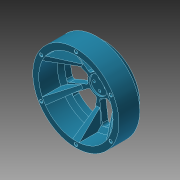
# Autodesk Inventor part: Переходник
Saved by Autodesk Inventor 2022 (Build 260153000, 153)
## iProperties
RuleStatus: InUse
Part Number: Переходник
Checked By: Якушев
Engr Approved By: Малов
Material: По умолчанию1
Document SubType Name: Modeling
Mfg Approved By: Судаков
Designer: Смирнов
Density: 1 g/cm^3
Appearance: Бирюзовый
AfterMaterialChange0: Материал
BeforeDocSave0: Материал
AfterAnyiPropertyChange0: Материал
Материал: По умолчанию1
Author: Смирнов
Autodesk Inventor part; units mm, degrees
ref_plane "YZ Plane" through (0, 0, 0) normal (1, 0, 0) x (0, 1, 0)
ref_plane "XZ Plane" through (0, 0, 0) normal (0, 1, 0) x (-1, 0, 0)
ref_plane "XY Plane" through (0, 0, 0) normal (0, 0, 1) x (1, 0, 0)
sketch "Эскиз1" plane through (0, 0, 0) normal (0, 0, 1) x (1, 0, 0)
  line L0 (0, 0) -> (0, 60)
  line L1 (0, 38) -> (0, 30)
  line L2 (0, 30) -> (45, 30)
  line L3 (50, 25) -> (50, 0)
  line L4 (50, 0) -> (58, 0)
  line L5 (58, 0) -> (58, 28)
  line L6 (48, 38) -> (0, 38)
  line L7 (45, 30) -> (50, 25)
  line L8 (48, 38) -> (58, 28)
  point P0 (50, 30)
  point P1 (58, 38)
  dimension "d0" = 100
  dimension "d1" = 116
  dimension "d2" = 8
  dimension "d3" = 30
  dimension "d4" = 5
  dimension "d5" = 5
  dimension "d6" = 10
  dimension "d7" = 10
  dimension "d36" = 8
  constraints: 18 end point, 6 point on line, 2 horizontal, 2 perpendicular, 1 midpoint, 1 vertical
  measures "d0" diameter of L3 L0
  measures "d1" diameter of L5 L0
  measures "d2" distance of L3.end L4.end
  measures "d3" distance of point (50, 30) L3.end
  measures "d4" distance of L2.end point (50, 30)
  measures "d5" distance of L3.start point (50, 30)
  measures "d6" distance of L6.start point (58, 38)
  measures "d7" distance of L5.end point (58, 38)
  measures "d36" distance between parallel lines of L2 L6
revolve "Вращение1" add sketch "Эскиз1" angle 360 about axis through (0, 0, 0) along (0, 1, 0)
sketch "Эскиз2" plane through (0, 0, 0) normal (1, 0, 0) x (0, 1, 0)
  line L0 (0, 50) -> (25, 50) projected
  line L1 (25, 50) -> (30, 45) projected
  line L2 (30, 45) -> (30, -45) projected
  line L3 (0, 50) -> (30, 25)
  line L4 (-5.8, 0) -> (34.8, 0) projected
  point P0 (0, 0)
  dimension "d9" = 25
  constraints: 2 end point, 1 point on line
  measures "d9" distance from line of L3.end L0
revolve "Вращение2" add sketch "Эскиз2" angle 10 mid plane about axis through (0, -10, 0) along (0, 1, 0)
pattern_circular "Круговой массив1" count 6 over 360 about axis through (0, 14, 0) along (0, -1, 0) of "Вращение2"
sketch "Эскиз3" plane through (0, 30, 0) normal (0, -1, 0) x (1, 0, 0)
  circle A0 centre (0, 0) radius 7.5 construction
  line L0 (0, 0) -> (0, 24.5029) construction
  circle A1 centre (0, 7.5) radius 1.7
  circle A2 centre (-7.5, 0) radius 1.7
  circle A3 centre (0, 0) radius 7.5 construction
  circle A4 centre (0, -7.5) radius 1.7
  circle A5 centre (0, 0) radius 7.5 construction
  circle A6 centre (7.5, 0) radius 1.7
  circle A7 centre (0, 0) radius 7.5 construction
  dimension "d19" = 15
  dimension "d14" = 3.4
  dimension "d17" = 360
  constraints: 4 centre point, 3 coincident, 2 end point, 2 horizontal alignment, 2 vertical alignment, 1 point on line, 1 vertical, 23 other
  measures "d14" diameter of A1
extrude "Выдавливание1" cut sketch "Эскиз3" against normal through all
sketch "Эскиз4" plane through (0, 30, 0) normal (0, -1, 0) x (1, 0, 0)
  circle A0 centre (0, 0) radius 12
  dimension "d22" = 24
  constraints: 1 centre point, 1 coincident
  measures "d22" diameter of A0
extrude "Выдавливание2" cut sketch "Эскиз4" against normal blind 2
sketch "Эскиз5" plane through (0, 30, 0) normal (0, -1, 0) x (1, 0, 0)
  arc A0 (40.7839, -19.0178) -> (40.7839, 19.0178) centre (0, 0) ccw projected
  circle A1 centre (0, 0) radius 12 construction
  circle A2 centre (0, 0) radius 14
  line L0 (0, 0) -> (41.5746, 17.2208)
  line L1 (0, 0) -> (72.7869, 0) construction
  line L2 (0, 0) -> (41.5746, -17.2208)
  point P0 (12.9343, -5.3576)
  point P1 (12.9343, 5.3576)
  dimension "d25" = 2
  dimension "d26" = 45
  constraints: 6 end point, 2 point on circle, 1 centre point, 1 coincident, 1 horizontal, 1 other
  measures "d25" radial gap between concentric circles of A2 A1
  measures "d26" angle of L2 L0
extrude "Выдавливание3" cut sketch "Эскиз5" against normal through all contours L2 A2 L0 A0
fillet "Сопряжение1" radius 3 4 edges at (12.9343, 34, 5.3576) (12.9343, 34, -5.3576) (41.5746, 34, 17.2208) (41.5746, 34, -17.2208)
pattern_circular "Круговой массив2" count 6 over 360 about axis through (0, 14, 0) along (0, -1, 0) of "Сопряжение1", "Выдавливание3"
chamfer "Фаска1" distance 2 angle 45 4 edges at (-1.7, 38, -7.5) (-9.2, 38, 0) (-1.7, 38, 7.5) (5.8, 38, 0)
sketch "Эскиз6" plane through (0, 0, 0) normal (0, -1, 0) x (1, 0, 0)
  line L0 (0, 0) -> (0, 75.0526) construction
  circle A0 centre (0, 0) radius 58 construction
  arc A1 (40.9576, 28.6788) -> (4.3578, 49.8097) centre (0, 0) ccw construction
  arc A2 (4.3578, 49.8097) -> (-4.3578, 49.8097) centre (0, 0) ccw construction
  circle A3 centre (0, 0) radius 58 construction
  arc A4 (-4.3578, 49.8097) -> (-40.9576, 28.6788) centre (0, 0) ccw construction
  arc A5 (4.3578, 49.8097) -> (-4.3578, 49.8097) centre (0, 0) ccw construction
  arc A6 (40.9576, 28.6788) -> (4.3578, 49.8097) centre (0, 0) ccw construction
  arc A7 (45.3154, 21.1309) -> (40.9576, 28.6788) centre (0, 0) ccw construction
  arc A8 (45.3154, -21.1309) -> (45.3154, 21.1309) centre (0, 0) ccw construction
  arc A9 (40.9576, -28.6788) -> (45.3154, -21.1309) centre (0, 0) ccw construction
  arc A10 (4.3578, -49.8097) -> (40.9576, -28.6788) centre (0, 0) ccw construction
  arc A11 (-4.3578, -49.8097) -> (4.3578, -49.8097) centre (0, 0) ccw construction
  arc A12 (-40.9576, -28.6788) -> (-4.3578, -49.8097) centre (0, 0) ccw construction
  arc A13 (-45.3154, -21.1309) -> (-40.9576, -28.6788) centre (0, 0) ccw construction
  arc A14 (-45.3154, 21.1309) -> (-45.3154, -21.1309) centre (0, 0) ccw construction
  arc A15 (-40.9576, 28.6788) -> (-45.3154, 21.1309) centre (0, 0) ccw construction
  line L1 (0, 58) -> (0, 50) construction
  point P0 (0, 54)
  constraints: 4 end point, 1 midpoint, 1 point on circle, 1 point on line, 1 vertical, 1 vertical alignment, 1 other
hole "Отверстие1" at (0, 0, 54) direction (0, 1, 0) diameter 3.9 depth 8 countersink diameter 4.5 countersink angle 90
pattern_circular "Круговой массив3" count 6 over 360 about axis through (0, 14, 0) along (0, -1, 0) of "Отверстие1"
sketch "Эскиз7" plane through (0, 38, 0) normal (0, 1, 0) x (1, 0, 0)
  line L0 (18.8219, 3.6597) -> (13.4444, 10.6677) construction
  line L1 (13.4444, 10.6677) -> (-8.0124, -5.7967) construction
  line L2 (-8.0124, -5.7967) -> (-2.6349, -12.8048) construction
  line L3 (-2.6349, -12.8048) -> (18.8219, 3.6597) construction
  line L4 (33.2357, 25.5027) -> (13.2753, 10.1865) projected
  point P0 (0, 0)
  constraints: 1 parallel, 2 other
equation "\"d5\" = d4"
equation "\"d6\" = d7"
